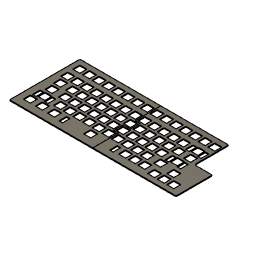
explore-rev3-plate-v1_full (Autodesk Fusion 360 design; units mm, degrees)
Autodesk Fusion 360 part; units mm, degrees
(part 1 of 4)
sketch "Sketch1" plane through (0, 0, 0) normal (0, 1, 0) x (1, 0, 0)
  line L0 (153.7375, -53.475) -> (166.7375, -53.475)
  line L1 (224.675, -92.075) -> (224.675, -105.075)
  line L2 (220.4125, -110.625) -> (233.4125, -110.625)
  line L3 (220.4125, -124.625) -> (233.4125, -124.625)
  line L4 (201.3625, -124.625) -> (214.3625, -124.625)
  line L5 (200.8625, -111.125) -> (200.8625, -124.125)
  line L6 (205.625, -92.075) -> (205.625, -105.075)
  line L7 (187.075, -91.575) -> (200.075, -91.575)
  arc A0 (201.3625, -110.625) -> (200.8625, -111.125) centre (201.3625, -111.125) ccw
  line L8 (219.625, -92.075) -> (219.625, -105.075)
  arc A1 (224.675, -105.075) -> (225.175, -105.575) centre (225.175, -105.075) ccw
  arc A2 (219.9125, -124.125) -> (220.4125, -124.625) centre (220.4125, -124.125) ccw
  line L9 (219.9125, -111.125) -> (219.9125, -124.125)
  line L10 (200.575, -92.075) -> (200.575, -105.075)
  line L11 (196.6, -72.525) -> (209.6, -72.525)
  line L12 (187.075, -105.575) -> (200.075, -105.575)
  line L13 (196.6, -86.525) -> (209.6, -86.525)
  line L14 (191.8375, -67.475) -> (204.8375, -67.475)
  line L15 (168.025, -91.575) -> (181.025, -91.575)
  arc A3 (172, -73.025) -> (171.5, -72.525) centre (171.5, -73.025) ccw
  arc A4 (166.7375, -67.475) -> (167.2375, -66.975) centre (166.7375, -66.975) ccw
  line L16 (177.55, -72.525) -> (190.55, -72.525)
  arc A5 (177.55, -72.525) -> (177.05, -73.025) centre (177.55, -73.025) ccw
  arc A6 (185.7875, -67.475) -> (186.2875, -66.975) centre (185.7875, -66.975) ccw
  arc A7 (171.5, -86.525) -> (172, -86.025) centre (171.5, -86.025) ccw
  arc A8 (196.6, -72.525) -> (196.1, -73.025) centre (196.6, -73.025) ccw
  line L17 (177.05, -73.025) -> (177.05, -86.025)
  arc A9 (191.3375, -66.975) -> (191.8375, -67.475) centre (191.8375, -66.975) ccw
  arc A10 (225.175, -91.575) -> (224.675, -92.075) centre (225.175, -92.075) ccw
  line L18 (215.65, -86.525) -> (228.65, -86.525)
  arc A11 (209.6, -86.525) -> (210.1, -86.025) centre (209.6, -86.025) ccw
  arc A12 (210.3875, -66.975) -> (210.8875, -67.475) centre (210.8875, -66.975) ccw
  arc A13 (215.15, -86.025) -> (215.65, -86.525) centre (215.65, -86.025) ccw
  arc A14 (200.575, -92.075) -> (200.075, -91.575) centre (200.075, -92.075) ccw
  arc A15 (215.65, -72.525) -> (215.15, -73.025) centre (215.65, -73.025) ccw
  line L19 (210.1, -73.025) -> (210.1, -86.025)
  line L20 (158.5, -72.525) -> (171.5, -72.525)
  arc A16 (234.2, -86.025) -> (234.7, -86.525) centre (234.7, -86.025) ccw
  line L21 (158.5, -86.525) -> (171.5, -86.525)
  arc A17 (162.475, -92.075) -> (161.975, -91.575) centre (161.975, -92.075) ccw
  arc A18 (233.9125, -11.1125) -> (233.4125, -10.6125) centre (233.4125, -11.1125) ccw
  arc A19 (214.8625, -34.925) -> (214.3625, -34.425) centre (214.3625, -34.925) ccw
  arc A20 (233.4125, -24.6125) -> (233.9125, -24.1125) centre (233.4125, -24.1125) ccw
  line L22 (195.8125, -11.1125) -> (195.8125, -24.1125)
  line L23 (233.9125, -11.1125) -> (233.9125, -24.1125)
  arc A21 (195.8125, -34.925) -> (195.3125, -34.425) centre (195.3125, -34.925) ccw
  line L24 (201.3625, -34.425) -> (214.3625, -34.425)
  line L25 (214.8625, -11.1125) -> (214.8625, -24.1125)
  arc A22 (214.8625, -11.1125) -> (214.3625, -10.6125) centre (214.3625, -11.1125) ccw
  arc A23 (200.8625, -24.1125) -> (201.3625, -24.6125) centre (201.3625, -24.1125) ccw
  arc A24 (220.4125, -10.6125) -> (219.9125, -11.1125) centre (220.4125, -11.1125) ccw
  line L26 (214.8625, -34.925) -> (214.8625, -47.925)
  line L27 (195.8125, -34.925) -> (195.8125, -47.925)
  line L28 (219.9125, -34.925) -> (219.9125, -47.925)
  line L29 (200.8625, -34.925) -> (200.8625, -47.925)
  line L30 (233.9125, -34.925) -> (233.9125, -47.925)
  arc A25 (205.625, -105.075) -> (206.125, -105.575) centre (206.125, -105.075) ccw
  line L31 (201.3625, -110.625) -> (214.3625, -110.625)
  line L32 (233.9125, -111.125) -> (233.9125, -124.125)
  line L33 (214.8625, -111.125) -> (214.8625, -124.125)
  arc A26 (214.3625, -124.625) -> (214.8625, -124.125) centre (214.3625, -124.125) ccw
  line L34 (206.125, -105.575) -> (219.125, -105.575)
  arc A27 (219.125, -105.575) -> (219.625, -105.075) centre (219.125, -105.075) ccw
  arc A28 (233.9125, -111.125) -> (233.4125, -110.625) centre (233.4125, -111.125) ccw
  arc A29 (200.8625, -124.125) -> (201.3625, -124.625) centre (201.3625, -124.125) ccw
  arc A30 (200.075, -105.575) -> (200.575, -105.075) centre (200.075, -105.075) ccw
  arc A31 (220.4125, -110.625) -> (219.9125, -111.125) centre (220.4125, -111.125) ccw
  arc A32 (233.4125, -124.625) -> (233.9125, -124.125) centre (233.4125, -124.125) ccw
  arc A33 (214.8625, -111.125) -> (214.3625, -110.625) centre (214.3625, -111.125) ccw
  line L35 (220.4125, -10.6125) -> (233.4125, -10.6125)
  arc A34 (214.3625, -24.6125) -> (214.8625, -24.1125) centre (214.3625, -24.1125) ccw
  arc A35 (219.9125, -24.1125) -> (220.4125, -24.6125) centre (220.4125, -24.1125) ccw
  line L36 (220.4125, -24.6125) -> (233.4125, -24.6125)
  line L37 (201.3625, -24.6125) -> (214.3625, -24.6125)
  arc A36 (201.3625, -34.425) -> (200.8625, -34.925) centre (201.3625, -34.925) ccw
  line L38 (200.8625, -11.1125) -> (200.8625, -24.1125)
  arc A37 (195.8125, -11.1125) -> (195.3125, -10.6125) centre (195.3125, -11.1125) ccw
  line L39 (201.3625, -10.6125) -> (214.3625, -10.6125)
  line L40 (220.4125, -34.425) -> (233.4125, -34.425)
  arc A38 (233.9125, -34.925) -> (233.4125, -34.425) centre (233.4125, -34.925) ccw
  line L41 (219.9125, -11.1125) -> (219.9125, -24.1125)
  arc A39 (201.3625, -10.6125) -> (200.8625, -11.1125) centre (201.3625, -11.1125) ccw
  arc A40 (220.4125, -34.425) -> (219.9125, -34.925) centre (220.4125, -34.925) ccw
  arc A41 (195.3125, -24.6125) -> (195.8125, -24.1125) centre (195.3125, -24.1125) ccw
  arc A42 (276.775, -115.8875) -> (276.275, -115.3875) centre (276.275, -115.8875) ccw
  line L42 (281.825, -115.8875) -> (281.825, -128.8875)
  arc A43 (143.425, -92.075) -> (142.925, -91.575) centre (142.925, -92.075) ccw
  line L43 (18.0063, -86.525) -> (31.0063, -86.525)
  arc A44 (10.8625, -10.6125) -> (10.3625, -11.1125) centre (10.8625, -11.1125) ccw
  arc A45 (29.9125, -10.6125) -> (29.4125, -11.1125) centre (29.9125, -11.1125) ccw
  arc A46 (148.975, -91.575) -> (148.475, -92.075) centre (148.975, -92.075) ccw
  arc A47 (10.3625, -24.1125) -> (10.8625, -24.6125) centre (10.8625, -24.1125) ccw
  arc A48 (42.9125, -24.6125) -> (43.4125, -24.1125) centre (42.9125, -24.1125) ccw
  line L44 (29.4125, -34.925) -> (29.4125, -47.925)
  line L45 (14.3308, -92.575) -> (20.3308, -92.575)
  arc A49 (152.95, -73.025) -> (152.45, -72.525) centre (152.45, -73.025) ccw
  line L46 (29.9125, -34.425) -> (42.9125, -34.425)
  line L47 (314.875, -115.8875) -> (314.875, -128.8875)
  line L48 (86.5625, -11.1125) -> (86.5625, -24.1125)
  arc A50 (13.8308, -107.075) -> (14.3308, -107.575) centre (14.3308, -107.075) ccw
  arc A51 (124.375, -92.075) -> (123.875, -91.575) centre (123.875, -92.075) ccw
  line L49 (10.8625, -10.6125) -> (23.8625, -10.6125)
  arc A52 (38.9375, -66.975) -> (39.4375, -67.475) centre (39.4375, -66.975) ccw
  line L50 (36.5563, -111.125) -> (36.5563, -124.125)
  line L51 (29.9125, -24.6125) -> (42.9125, -24.6125)
  line L52 (29.9125, -10.6125) -> (42.9125, -10.6125)
  arc A53 (115.1375, -66.975) -> (115.6375, -67.475) centre (115.6375, -66.975) ccw
  arc A54 (10.8625, -34.425) -> (10.3625, -34.925) centre (10.8625, -34.925) ccw
  line L53 (91.825, -105.575) -> (104.825, -105.575)
  arc A55 (29.9125, -34.425) -> (29.4125, -34.925) centre (29.9125, -34.925) ccw
  arc A56 (109.5875, -67.475) -> (110.0875, -66.975) centre (109.5875, -66.975) ccw
  arc A57 (24.3625, -34.925) -> (23.8625, -34.425) centre (23.8625, -34.925) ccw
  line L54 (53.725, -105.575) -> (66.725, -105.575)
  arc A58 (50.0563, -124.625) -> (50.5563, -124.125) centre (50.0563, -124.125) ccw
  line L55 (43.4125, -34.925) -> (43.4125, -47.925)
  arc A59 (20.8308, -93.075) -> (20.3308, -92.575) centre (20.3308, -93.075) ccw
  arc A60 (110.0875, -53.975) -> (109.5875, -53.475) centre (109.5875, -53.975) ccw
  arc A61 (48.9625, -34.425) -> (48.4625, -34.925) centre (48.9625, -34.925) ccw
  arc A62 (92.3063, -112.125) -> (91.8063, -111.625) centre (91.8063, -112.125) ccw
  arc A63 (48.9625, -10.6125) -> (48.4625, -11.1125) centre (48.9625, -11.1125) ccw
  arc A64 (43.7, -86.025) -> (44.2, -86.525) centre (44.2, -86.025) ccw
  arc A65 (134.1875, -66.975) -> (134.6875, -67.475) centre (134.6875, -66.975) ccw
  arc A66 (43.4125, -11.1125) -> (42.9125, -10.6125) centre (42.9125, -11.1125) ccw
  arc A67 (147.6875, -67.475) -> (148.1875, -66.975) centre (147.6875, -66.975) ccw
  line L56 (120.4, -86.525) -> (133.4, -86.525)
  line L57 (29.4125, -11.1125) -> (29.4125, -24.1125)
  arc A68 (114.35, -86.525) -> (114.85, -86.025) centre (114.35, -86.025) ccw
  arc A69 (96.0875, -66.975) -> (96.5875, -67.475) centre (96.5875, -66.975) ccw
  arc A70 (138.95, -86.025) -> (139.45, -86.525) centre (139.45, -86.025) ccw
  line L58 (48.4625, -11.1125) -> (48.4625, -24.1125)
  arc A71 (20.3308, -107.575) -> (20.8308, -107.075) centre (20.3308, -107.075) ccw
  line L59 (14.3308, -107.575) -> (20.3308, -107.575)
  arc A72 (26.2438, -124.625) -> (26.7438, -124.125) centre (26.2438, -124.125) ccw
  line L60 (13.2438, -110.625) -> (26.2438, -110.625)
  line L61 (22.7688, -91.575) -> (35.7688, -91.575)
  arc A73 (43.4125, -34.925) -> (42.9125, -34.425) centre (42.9125, -34.925) ccw
  arc A74 (31.5063, -73.025) -> (31.0063, -72.525) centre (31.0063, -73.025) ccw
  arc A75 (36.2688, -92.075) -> (35.7688, -91.575) centre (35.7688, -92.075) ccw
  line L62 (85.3063, -112.125) -> (85.3063, -126.125)
  arc A76 (314.875, -115.8875) -> (314.375, -115.3875) centre (314.375, -115.8875) ccw
  line L63 (50.5563, -111.125) -> (50.5563, -124.125)
  arc A77 (153.2375, -66.975) -> (153.7375, -67.475) centre (153.7375, -66.975) ccw
  arc A78 (91.325, -105.075) -> (91.825, -105.575) centre (91.825, -105.075) ccw
  line L64 (24.3625, -11.1125) -> (24.3625, -24.1125)
  arc A79 (18.0063, -72.525) -> (17.5063, -73.025) centre (18.0063, -73.025) ccw
  arc A80 (12.7438, -124.125) -> (13.2438, -124.625) centre (13.2438, -124.125) ccw
  line L65 (12.7438, -111.125) -> (12.7438, -124.125)
  line L66 (114.85, -73.025) -> (114.85, -86.025)
  line L67 (272.8, -67.475) -> (285.8, -67.475)
  arc A81 (119.6125, -11.1125) -> (119.1125, -10.6125) centre (119.1125, -11.1125) ccw
  arc A82 (277.0625, -24.1125) -> (277.5625, -24.6125) centre (277.5625, -24.1125) ccw
  arc A83 (266.0995, -35.925) -> (265.5995, -35.425) centre (265.5995, -35.925) ccw
  line L68 (53.225, -92.075) -> (53.225, -105.075)
  line L69 (281.0943, -73.525) -> (287.0943, -73.525)
  line L70 (91.325, -92.075) -> (91.325, -105.075)
  arc A84 (281.0943, -73.525) -> (280.5943, -74.025) centre (281.0943, -74.025) ccw
  arc A85 (272.3, -66.975) -> (272.8, -67.475) centre (272.8, -66.975) ccw
  line L71 (277.0625, -11.1125) -> (277.0625, -24.1125)
  line L72 (152.95, -73.025) -> (152.95, -86.025)
  arc A86 (157.2125, -24.6125) -> (157.7125, -24.1125) centre (157.2125, -24.1125) ccw
  arc A87 (290.5625, -24.6125) -> (291.0625, -24.1125) centre (290.5625, -24.1125) ccw
  arc A88 (87.0625, -34.425) -> (86.5625, -34.925) centre (87.0625, -34.925) ccw
  arc A89 (128.6375, -67.475) -> (129.1375, -66.975) centre (128.6375, -66.975) ccw
  arc A90 (15.625, -53.475) -> (15.125, -53.975) centre (15.625, -53.975) ccw
  line L73 (250.8688, -92.075) -> (250.8688, -105.075)
  arc A91 (285.8, -67.475) -> (286.3, -66.975) centre (285.8, -66.975) ccw
  line L74 (279.1563, -73.025) -> (279.1563, -86.025)
  line L75 (272.0125, -11.1125) -> (272.0125, -24.1125)
  arc A92 (272.0125, -11.1125) -> (271.5125, -10.6125) centre (271.5125, -11.1125) ccw
  line L76 (144.2125, -10.6125) -> (157.2125, -10.6125)
  line L77 (131.8063, -111.125) -> (131.8063, -124.125)
  line L78 (287.5943, -74.025) -> (287.5943, -88.025)
  arc A93 (158.5, -72.525) -> (158, -73.025) centre (158.5, -73.025) ccw
  line L79 (67.5125, -11.1125) -> (67.5125, -24.1125)
  line L80 (125.1625, -24.6125) -> (138.1625, -24.6125)
  arc A94 (158, -86.025) -> (158.5, -86.525) centre (158.5, -86.025) ccw
  line L81 (96.5875, -53.475) -> (109.5875, -53.475)
  line L82 (119.6125, -11.1125) -> (119.6125, -24.1125)
  line L83 (81.5125, -11.1125) -> (81.5125, -24.1125)
  line L84 (145.8063, -111.125) -> (145.8063, -124.125)
  arc A95 (29.125, -53.975) -> (28.625, -53.475) centre (28.625, -53.975) ccw
  line L85 (280.5943, -74.025) -> (280.5943, -88.025)
  line L86 (124.6625, -11.1125) -> (124.6625, -24.1125)
  arc A96 (278.6563, -86.525) -> (279.1563, -86.025) centre (278.6563, -86.025) ccw
  line L87 (68.0125, -10.6125) -> (81.0125, -10.6125)
  line L88 (44.7068, -93.075) -> (44.7068, -107.075)
  line L89 (132.3063, -110.625) -> (145.3063, -110.625)
  arc A97 (124.6625, -24.1125) -> (125.1625, -24.6125) centre (125.1625, -24.1125) ccw
  line L90 (39.4375, -53.475) -> (52.4375, -53.475)
  arc A98 (279.1563, -73.025) -> (278.6563, -72.525) centre (278.6563, -73.025) ccw
  arc A99 (138.6625, -34.925) -> (138.1625, -34.425) centre (138.1625, -34.925) ccw
  arc A100 (23.8625, -48.425) -> (24.3625, -47.925) centre (23.8625, -47.925) ccw
  line L91 (72.275, -92.075) -> (72.275, -105.075)
  arc A101 (289.9755, -35.925) -> (289.4755, -35.425) centre (289.4755, -35.925) ccw
  arc A102 (100.0625, -48.425) -> (100.5625, -47.925) centre (100.0625, -47.925) ccw
  line L92 (125.1625, -10.6125) -> (138.1625, -10.6125)
  arc A103 (106.1125, -10.6125) -> (105.6125, -11.1125) centre (106.1125, -11.1125) ccw
  arc A104 (119.1125, -24.6125) -> (119.6125, -24.1125) centre (119.1125, -24.1125) ccw
  line L93 (281.825, -96.8375) -> (281.825, -109.8375)
  line L94 (87.0625, -48.425) -> (100.0625, -48.425)
  line L95 (129.925, -105.575) -> (142.925, -105.575)
  arc A105 (100.5625, -34.925) -> (100.0625, -34.425) centre (100.0625, -34.925) ccw
  line L96 (110.375, -92.075) -> (110.375, -105.075)
  arc A106 (115.6375, -53.475) -> (115.1375, -53.975) centre (115.6375, -53.975) ccw
  line L97 (105.6125, -34.925) -> (105.6125, -47.925)
  arc A107 (157.7125, -11.1125) -> (157.2125, -10.6125) centre (157.2125, -11.1125) ccw
  line L98 (143.425, -92.075) -> (143.425, -105.075)
  arc A108 (280.5943, -88.025) -> (281.0943, -88.525) centre (281.0943, -88.025) ccw
  arc A109 (287.5943, -74.025) -> (287.0943, -73.525) centre (287.0943, -74.025) ccw
  line L99 (295.825, -96.8375) -> (295.825, -109.8375)
  arc A110 (144.2125, -34.425) -> (143.7125, -34.925) centre (144.2125, -34.925) ccw
  arc A111 (133.4, -86.525) -> (133.9, -86.025) centre (133.4, -86.025) ccw
  arc A112 (39.4375, -53.475) -> (38.9375, -53.975) centre (39.4375, -53.975) ccw
  arc A113 (129.425, -105.075) -> (129.925, -105.575) centre (129.925, -105.075) ccw
  line L100 (282.325, -129.3875) -> (295.325, -129.3875)
  arc A114 (87.0625, -10.6125) -> (86.5625, -11.1125) centre (87.0625, -11.1125) ccw
  line L101 (10.8625, -48.425) -> (23.8625, -48.425)
  line L102 (138.6625, -34.925) -> (138.6625, -47.925)
  line L103 (20.8308, -93.075) -> (20.8308, -107.075)
  arc A115 (86.5625, -24.1125) -> (87.0625, -24.6125) centre (87.0625, -24.1125) ccw
  arc A116 (42.9125, -48.425) -> (43.4125, -47.925) centre (42.9125, -47.925) ccw
  line L104 (129.925, -91.575) -> (142.925, -91.575)
  arc A117 (100.5625, -11.1125) -> (100.0625, -10.6125) centre (100.0625, -11.1125) ccw
  line L105 (48.4625, -34.925) -> (48.4625, -47.925)
  line L106 (282.325, -110.3375) -> (295.325, -110.3375)
  line L107 (157.7125, -11.1125) -> (157.7125, -24.1125)
  arc A118 (287.0943, -88.525) -> (287.5943, -88.025) centre (287.0943, -88.025) ccw
  line L108 (300.875, -115.8875) -> (300.875, -128.8875)
  arc A119 (125.1625, -10.6125) -> (124.6625, -11.1125) centre (125.1625, -11.1125) ccw
  line L109 (133.9, -73.025) -> (133.9, -86.025)
  arc A120 (132.3063, -110.625) -> (131.8063, -111.125) centre (132.3063, -111.125) ccw
  arc A121 (10.3625, -47.925) -> (10.8625, -48.425) centre (10.8625, -47.925) ccw
  arc A122 (48.4625, -47.925) -> (48.9625, -48.425) centre (48.9625, -47.925) ccw
  line L110 (138.6625, -11.1125) -> (138.6625, -24.1125)
  arc A123 (133.9, -73.025) -> (133.4, -72.525) centre (133.4, -73.025) ccw
  arc A124 (91.0375, -53.975) -> (90.5375, -53.475) centre (90.5375, -53.975) ccw
  arc A125 (125.1625, -34.425) -> (124.6625, -34.925) centre (125.1625, -34.925) ccw
  line L111 (132.3063, -124.625) -> (145.3063, -124.625)
  line L112 (301.375, -115.3875) -> (314.375, -115.3875)
  line L113 (15.625, -53.475) -> (28.625, -53.475)
  arc A126 (123.875, -105.575) -> (124.375, -105.075) centre (123.875, -105.075) ccw
  arc A127 (96.5875, -53.475) -> (96.0875, -53.975) centre (96.5875, -53.975) ccw
  arc A128 (142.925, -105.575) -> (143.425, -105.075) centre (142.925, -105.075) ccw
  arc A129 (157.7125, -34.925) -> (157.2125, -34.425) centre (157.2125, -34.925) ccw
  line L114 (29.9125, -48.425) -> (42.9125, -48.425)
  line L115 (143.7125, -11.1125) -> (143.7125, -24.1125)
  line L116 (48.9625, -10.6125) -> (61.9625, -10.6125)
  line L117 (281.0943, -88.525) -> (287.0943, -88.525)
  line L118 (100.5625, -11.1125) -> (100.5625, -24.1125)
  line L119 (295.825, -115.8875) -> (295.825, -128.8875)
  arc A130 (314.375, -129.3875) -> (314.875, -128.8875) centre (314.375, -128.8875) ccw
  line L120 (87.0625, -24.6125) -> (100.0625, -24.6125)
  line L121 (119.6125, -34.925) -> (119.6125, -47.925)
  arc A131 (295.325, -110.3375) -> (295.825, -109.8375) centre (295.325, -109.8375) ccw
  line L122 (157.7125, -34.925) -> (157.7125, -47.925)
  arc A132 (144.2125, -10.6125) -> (143.7125, -11.1125) centre (144.2125, -11.1125) ccw
  arc A133 (281.825, -109.8375) -> (282.325, -110.3375) centre (282.325, -109.8375) ccw
  arc A134 (86.5625, -47.925) -> (87.0625, -48.425) centre (87.0625, -47.925) ccw
  line L123 (37.7068, -93.075) -> (37.7068, -107.075)
  line L124 (105.6125, -11.1125) -> (105.6125, -24.1125)
  line L125 (134.6875, -67.475) -> (147.6875, -67.475)
  arc A135 (145.3063, -124.625) -> (145.8063, -124.125) centre (145.3063, -124.125) ccw
  arc A136 (276.275, -129.3875) -> (276.775, -128.8875) centre (276.275, -128.8875) ccw
  line L126 (86.5625, -34.925) -> (86.5625, -47.925)
  arc A137 (145.8063, -111.125) -> (145.3063, -110.625) centre (145.3063, -111.125) ccw
  arc A138 (106.1125, -34.425) -> (105.6125, -34.925) centre (106.1125, -34.925) ccw
  arc A139 (143.7125, -24.1125) -> (144.2125, -24.6125) centre (144.2125, -24.1125) ccw
  arc A140 (29.4125, -47.925) -> (29.9125, -48.425) centre (29.9125, -47.925) ccw
  arc A141 (295.825, -96.8375) -> (295.325, -96.3375) centre (295.325, -96.8375) ccw
  arc A142 (148.475, -105.075) -> (148.975, -105.575) centre (148.975, -105.075) ccw
  arc A143 (131.8063, -124.125) -> (132.3063, -124.625) centre (132.3063, -124.125) ccw
  line L127 (124.6625, -34.925) -> (124.6625, -47.925)
  line L128 (24.3625, -34.925) -> (24.3625, -47.925)
  line L129 (67.225, -92.075) -> (67.225, -105.075)
  line L130 (139.45, -72.525) -> (152.45, -72.525)
  line L131 (158, -73.025) -> (158, -86.025)
  arc A144 (295.325, -129.3875) -> (295.825, -128.8875) centre (295.325, -128.8875) ccw
  arc A145 (86.275, -92.075) -> (85.775, -91.575) centre (85.775, -92.075) ccw
  arc A146 (105.6125, -24.1125) -> (106.1125, -24.6125) centre (106.1125, -24.1125) ccw
  arc A147 (110.875, -91.575) -> (110.375, -92.075) centre (110.875, -92.075) ccw
  line L132 (85.8063, -111.625) -> (91.8063, -111.625)
  line L133 (100.5625, -34.925) -> (100.5625, -47.925)
  arc A148 (100.0625, -24.6125) -> (100.5625, -24.1125) centre (100.0625, -24.1125) ccw
  arc A149 (120.4, -72.525) -> (119.9, -73.025) centre (120.4, -73.025) ccw
  line L134 (13.8308, -93.075) -> (13.8308, -107.075)
  arc A150 (85.8063, -111.625) -> (85.3063, -112.125) centre (85.8063, -112.125) ccw
  line L135 (85.8063, -126.625) -> (91.8063, -126.625)
  line L136 (301.375, -129.3875) -> (314.375, -129.3875)
  arc A151 (300.875, -128.8875) -> (301.375, -129.3875) centre (301.375, -128.8875) ccw
  arc A152 (23.8625, -24.6125) -> (24.3625, -24.1125) centre (23.8625, -24.1125) ccw
  arc A153 (105.6125, -47.925) -> (106.1125, -48.425) centre (106.1125, -47.925) ccw
  arc A154 (85.3063, -126.125) -> (85.8063, -126.625) centre (85.8063, -126.125) ccw
  arc A155 (295.825, -115.8875) -> (295.325, -115.3875) centre (295.325, -115.8875) ccw
  arc A156 (281.825, -128.8875) -> (282.325, -129.3875) centre (282.325, -128.8875) ccw
  arc A157 (301.375, -115.3875) -> (300.875, -115.8875) centre (301.375, -115.8875) ccw
  arc A158 (110.375, -105.075) -> (110.875, -105.575) centre (110.875, -105.075) ccw
  arc A159 (282.325, -115.3875) -> (281.825, -115.8875) centre (282.325, -115.8875) ccw
  line L137 (22.2688, -92.075) -> (22.2688, -105.075)
  line L138 (36.2688, -92.075) -> (36.2688, -105.075)
  arc A160 (91.8063, -126.625) -> (92.3063, -126.125) centre (91.8063, -126.125) ccw
  arc A161 (104.825, -105.575) -> (105.325, -105.075) centre (104.825, -105.075) ccw
  arc A162 (139.45, -72.525) -> (138.95, -73.025) centre (139.45, -73.025) ccw
  line L139 (10.3625, -34.925) -> (10.3625, -47.925)
  line L140 (92.3063, -112.125) -> (92.3063, -126.125)
  arc A163 (129.925, -91.575) -> (129.425, -92.075) centre (129.925, -92.075) ccw
  line L141 (276.775, -115.8875) -> (276.775, -128.8875)
  arc A164 (85.775, -105.575) -> (86.275, -105.075) centre (85.775, -105.075) ccw
  line L142 (87.0625, -10.6125) -> (100.0625, -10.6125)
  line L143 (143.7125, -34.925) -> (143.7125, -47.925)
  line L144 (87.0625, -34.425) -> (100.0625, -34.425)
  line L145 (282.325, -115.3875) -> (295.325, -115.3875)
  arc A165 (36.5563, -124.125) -> (37.0563, -124.625) centre (37.0563, -124.125) ccw
  arc A166 (119.9, -86.025) -> (120.4, -86.525) centre (120.4, -86.025) ccw
  line L146 (60.8688, -110.625) -> (73.8688, -110.625)
  line L147 (101.35, -72.525) -> (114.35, -72.525)
  line L148 (10.8625, -24.6125) -> (23.8625, -24.6125)
  line L149 (17.5063, -73.025) -> (17.5063, -86.025)
  line L150 (10.3625, -11.1125) -> (10.3625, -24.1125)
  arc A167 (22.2688, -105.075) -> (22.7688, -105.575) centre (22.7688, -105.075) ccw
  line L151 (15.625, -67.475) -> (28.625, -67.475)
  line L152 (31.5063, -73.025) -> (31.5063, -86.025)
  arc A168 (15.125, -66.975) -> (15.625, -67.475) centre (15.625, -66.975) ccw
  arc A169 (44.2, -72.525) -> (43.7, -73.025) centre (44.2, -73.025) ccw
  line L153 (43.4125, -11.1125) -> (43.4125, -24.1125)
  arc A170 (44.2068, -107.575) -> (44.7068, -107.075) centre (44.2068, -107.075) ccw
  arc A171 (38.2068, -92.575) -> (37.7068, -93.075) centre (38.2068, -93.075) ccw
  arc A172 (91.825, -91.575) -> (91.325, -92.075) centre (91.825, -92.075) ccw
  arc A173 (60.3688, -124.125) -> (60.8688, -124.625) centre (60.8688, -124.125) ccw
  line L154 (101.35, -86.525) -> (114.35, -86.525)
  arc A174 (48.4625, -24.1125) -> (48.9625, -24.6125) centre (48.9625, -24.1125) ccw
  line L155 (96.5875, -67.475) -> (109.5875, -67.475)
  arc A175 (105.325, -92.075) -> (104.825, -91.575) centre (104.825, -92.075) ccw
  arc A176 (37.0563, -110.625) -> (36.5563, -111.125) centre (37.0563, -111.125) ccw
  line L156 (18.0063, -72.525) -> (31.0063, -72.525)
  arc A177 (35.7688, -105.575) -> (36.2688, -105.075) centre (35.7688, -105.075) ccw
  line L157 (60.3688, -111.125) -> (60.3688, -124.125)
  arc A178 (24.3625, -11.1125) -> (23.8625, -10.6125) centre (23.8625, -11.1125) ccw
  arc A179 (26.7438, -111.125) -> (26.2438, -110.625) centre (26.2438, -111.125) ccw
  arc A180 (29.4125, -24.1125) -> (29.9125, -24.6125) centre (29.9125, -24.1125) ccw
  arc A181 (13.2438, -110.625) -> (12.7438, -111.125) centre (13.2438, -111.125) ccw
  arc A182 (31.0063, -86.525) -> (31.5063, -86.025) centre (31.0063, -86.025) ccw
  line L158 (26.7438, -111.125) -> (26.7438, -124.125)
  arc A183 (14.3308, -92.575) -> (13.8308, -93.075) centre (14.3308, -93.075) ccw
  line L159 (38.2068, -107.575) -> (44.2068, -107.575)
  line L160 (43.7, -73.025) -> (43.7, -86.025)
  arc A184 (44.7068, -93.075) -> (44.2068, -92.575) centre (44.2068, -93.075) ccw
  line L161 (38.2068, -92.575) -> (44.2068, -92.575)
  arc A185 (50.5563, -111.125) -> (50.0563, -110.625) centre (50.0563, -111.125) ccw
  arc A186 (90.5375, -67.475) -> (91.0375, -66.975) centre (90.5375, -66.975) ccw
  line L162 (22.7688, -105.575) -> (35.7688, -105.575)
  arc A187 (17.5063, -86.025) -> (18.0063, -86.525) centre (18.0063, -86.025) ccw
  arc A188 (72.275, -105.075) -> (72.775, -105.575) centre (72.775, -105.075) ccw
  arc A189 (60.8688, -110.625) -> (60.3688, -111.125) centre (60.8688, -111.125) ccw
  arc A190 (53.225, -105.075) -> (53.725, -105.575) centre (53.725, -105.075) ccw
  arc A191 (74.3688, -111.125) -> (73.8688, -110.625) centre (73.8688, -111.125) ccw
  arc A192 (28.625, -67.475) -> (29.125, -66.975) centre (28.625, -66.975) ccw
  arc A193 (22.7688, -91.575) -> (22.2688, -92.075) centre (22.7688, -92.075) ccw
  arc A194 (101.35, -72.525) -> (100.85, -73.025) centre (101.35, -73.025) ccw
  line L163 (95.8, -73.025) -> (95.8, -86.025)
  line L164 (100.85, -73.025) -> (100.85, -86.025)
  arc A195 (114.85, -73.025) -> (114.35, -72.525) centre (114.35, -73.025) ccw
  arc A196 (66.725, -105.575) -> (67.225, -105.075) centre (66.725, -105.075) ccw
  arc A197 (73.8688, -124.625) -> (74.3688, -124.125) centre (73.8688, -124.125) ccw
  line L165 (91.825, -91.575) -> (104.825, -91.575)
  line L166 (60.8688, -124.625) -> (73.8688, -124.625)
  line L167 (13.2438, -124.625) -> (26.2438, -124.625)
  arc A198 (95.3, -86.525) -> (95.8, -86.025) centre (95.3, -86.025) ccw
  arc A199 (95.8, -73.025) -> (95.3, -72.525) centre (95.3, -73.025) ccw
  line L168 (10.8625, -34.425) -> (23.8625, -34.425)
  arc A200 (37.7068, -107.075) -> (38.2068, -107.575) centre (38.2068, -107.075) ccw
  line L169 (74.3688, -111.125) -> (74.3688, -124.125)
  arc A201 (100.85, -86.025) -> (101.35, -86.525) centre (101.35, -86.025) ccw
  line L170 (210.8875, -53.475) -> (223.8875, -53.475)
  line L171 (220.4125, -48.425) -> (233.4125, -48.425)
  arc A202 (195.3125, -48.425) -> (195.8125, -47.925) centre (195.3125, -47.925) ccw
  arc A203 (224.3875, -53.975) -> (223.8875, -53.475) centre (223.8875, -53.975) ccw
  arc A204 (229.9375, -53.475) -> (229.4375, -53.975) centre (229.9375, -53.975) ccw
  arc A205 (200.8625, -47.925) -> (201.3625, -48.425) centre (201.3625, -47.925) ccw
  arc A206 (219.9125, -47.925) -> (220.4125, -48.425) centre (220.4125, -47.925) ccw
  arc A207 (210.8875, -53.475) -> (210.3875, -53.975) centre (210.8875, -53.975) ccw
  arc A208 (205.3375, -53.975) -> (204.8375, -53.475) centre (204.8375, -53.975) ccw
  arc A209 (214.3625, -48.425) -> (214.8625, -47.925) centre (214.3625, -47.925) ccw
  line L172 (148.975, -91.575) -> (161.975, -91.575)
  arc A210 (233.4125, -48.425) -> (233.9125, -47.925) centre (233.4125, -47.925) ccw
  line L173 (201.3625, -48.425) -> (214.3625, -48.425)
  arc A211 (185.8063, -111.625) -> (185.3063, -112.125) centre (185.8063, -112.125) ccw
  arc A212 (167.525, -105.075) -> (168.025, -105.575) centre (168.025, -105.075) ccw
  line L174 (185.3063, -112.125) -> (185.3063, -126.125)
  arc A213 (192.3063, -112.125) -> (191.8063, -111.625) centre (191.8063, -112.125) ccw
  line L175 (185.8063, -126.625) -> (191.8063, -126.625)
  line L176 (268.0375, -34.425) -> (281.0375, -34.425)
  arc A214 (57.7, -73.025) -> (57.2, -72.525) centre (57.2, -73.025) ccw
  arc A215 (282.325, -96.3375) -> (281.825, -96.8375) centre (282.325, -96.8375) ccw
  arc A216 (81.0125, -24.6125) -> (81.5125, -24.1125) centre (81.0125, -24.1125) ccw
  arc A217 (238.9625, -124.125) -> (239.4625, -124.625) centre (239.4625, -124.125) ccw
  line L177 (282.325, -96.3375) -> (295.325, -96.3375)
  line L178 (105.325, -92.075) -> (105.325, -105.075)
  line L179 (252.9625, -34.925) -> (252.9625, -47.925)
  arc A218 (239.4625, -110.625) -> (238.9625, -111.125) centre (239.4625, -111.125) ccw
  line L180 (81.5125, -34.925) -> (81.5125, -47.925)
  arc A219 (252.4625, -124.625) -> (252.9625, -124.125) centre (252.4625, -124.125) ccw
  line L181 (239.4625, -110.625) -> (252.4625, -110.625)
  line L182 (129.425, -92.075) -> (129.425, -105.075)
  arc A220 (67.5125, -47.925) -> (68.0125, -48.425) centre (68.0125, -47.925) ccw
  line L183 (239.4625, -124.625) -> (252.4625, -124.625)
  arc A221 (77.5375, -53.475) -> (77.0375, -53.975) centre (77.5375, -53.975) ccw
  line L184 (238.9625, -111.125) -> (238.9625, -124.125)
  arc A222 (81.8, -86.025) -> (82.3, -86.525) centre (82.3, -86.025) ccw
  line L185 (81.8, -73.025) -> (81.8, -86.025)
  line L186 (48.9625, -24.6125) -> (61.9625, -24.6125)
  arc A223 (61.9625, -24.6125) -> (62.4625, -24.1125) centre (61.9625, -24.1125) ccw
  arc A224 (138.6625, -11.1125) -> (138.1625, -10.6125) centre (138.1625, -11.1125) ccw
  line L187 (138.95, -73.025) -> (138.95, -86.025)
  line L188 (264.8688, -92.075) -> (264.8688, -105.075)
  line L189 (48.9625, -48.425) -> (61.9625, -48.425)
  line L190 (277.5625, -10.6125) -> (290.5625, -10.6125)
  arc A225 (68.0125, -10.6125) -> (67.5125, -11.1125) centre (68.0125, -11.1125) ccw
  line L191 (120.4, -72.525) -> (133.4, -72.525)
  arc A226 (119.6125, -34.925) -> (119.1125, -34.425) centre (119.1125, -34.925) ccw
  line L192 (291.0625, -11.1125) -> (291.0625, -24.1125)
  line L193 (238.675, -92.075) -> (238.675, -105.075)
  arc A227 (283.4755, -35.425) -> (282.9755, -35.925) centre (283.4755, -35.925) ccw
  arc A228 (252.9625, -111.125) -> (252.4625, -110.625) centre (252.4625, -111.125) ccw
  line L194 (44.2, -86.525) -> (57.2, -86.525)
  line L195 (148.475, -92.075) -> (148.475, -105.075)
  line L196 (277.5625, -24.6125) -> (290.5625, -24.6125)
  arc A229 (63.25, -72.525) -> (62.75, -73.025) centre (63.25, -73.025) ccw
  line L197 (139.45, -86.525) -> (152.45, -86.525)
  line L198 (48.9625, -34.425) -> (61.9625, -34.425)
  line L199 (144.2125, -34.425) -> (157.2125, -34.425)
  arc A230 (238.175, -105.575) -> (238.675, -105.075) centre (238.175, -105.075) ccw
  line L200 (252.9625, -111.125) -> (252.9625, -124.125)
  arc A231 (277.5625, -10.6125) -> (277.0625, -11.1125) centre (277.5625, -11.1125) ccw
  arc A232 (271.5125, -24.6125) -> (272.0125, -24.1125) centre (271.5125, -24.1125) ccw
  line L201 (281.5375, -34.925) -> (281.5375, -47.925)
  line L202 (124.375, -92.075) -> (124.375, -105.075)
  line L203 (251.3688, -105.575) -> (264.3688, -105.575)
  line L204 (283.4755, -35.425) -> (289.4755, -35.425)
  arc A233 (138.1625, -24.6125) -> (138.6625, -24.1125) centre (138.1625, -24.1125) ccw
  line L205 (115.6375, -53.475) -> (128.6375, -53.475)
  line L206 (119.9, -73.025) -> (119.9, -86.025)
  arc A234 (81.5125, -34.925) -> (81.0125, -34.425) centre (81.0125, -34.925) ccw
  line L207 (68.0125, -34.425) -> (81.0125, -34.425)
  arc A235 (291.0625, -11.1125) -> (290.5625, -10.6125) centre (290.5625, -11.1125) ccw
  arc A236 (68.0125, -34.425) -> (67.5125, -34.925) centre (68.0125, -34.925) ccw
  arc A237 (281.5375, -34.925) -> (281.0375, -34.425) centre (281.0375, -34.925) ccw
  arc A238 (81.0125, -48.425) -> (81.5125, -47.925) centre (81.0125, -47.925) ccw
  arc A239 (81.5125, -11.1125) -> (81.0125, -10.6125) centre (81.0125, -11.1125) ccw
  arc A240 (264.3688, -105.575) -> (264.8688, -105.075) centre (264.3688, -105.075) ccw
  line L208 (144.2125, -24.6125) -> (157.2125, -24.6125)
  arc A241 (61.9625, -48.425) -> (62.4625, -47.925) centre (61.9625, -47.925) ccw
  arc A242 (268.0375, -34.425) -> (267.5375, -34.925) centre (268.0375, -34.925) ccw
  line L209 (125.1625, -34.425) -> (138.1625, -34.425)
  line L210 (172.2875, -53.975) -> (172.2875, -66.975)
  arc A243 (238.675, -92.075) -> (238.175, -91.575) centre (238.175, -92.075) ccw
  arc A244 (251.3688, -91.575) -> (250.8688, -92.075) centre (251.3688, -92.075) ccw
  line L211 (248.9875, -53.475) -> (261.9875, -53.475)
  line L212 (248.9875, -67.475) -> (261.9875, -67.475)
  arc A245 (72.775, -91.575) -> (72.275, -92.075) centre (72.775, -92.075) ccw
  line L213 (153.2375, -53.975) -> (153.2375, -66.975)
  line L214 (15.125, -53.975) -> (15.125, -66.975)
  line L215 (265.6563, -86.525) -> (278.6563, -86.525)
  line L216 (259.5995, -35.425) -> (265.5995, -35.425)
  line L217 (259.5995, -50.425) -> (265.5995, -50.425)
  line L218 (0, -140) -> (0, 0)
  line L219 (256.7183, -74.025) -> (256.7183, -88.025)
  line L220 (239.4625, -48.425) -> (252.4625, -48.425)
  arc A246 (264.8688, -92.075) -> (264.3688, -91.575) centre (264.3688, -92.075) ccw
  line L221 (129.1375, -53.975) -> (129.1375, -66.975)
  line L222 (110.875, -105.575) -> (123.875, -105.575)
  arc A247 (263.2183, -88.525) -> (263.7183, -88.025) centre (263.2183, -88.025) ccw
  line L223 (52.9375, -53.975) -> (52.9375, -66.975)
  arc A248 (263.7183, -74.025) -> (263.2183, -73.525) centre (263.2183, -74.025) ccw
  line L224 (37.0563, -124.625) -> (50.0563, -124.625)
  line L225 (191.3375, -53.975) -> (191.3375, -66.975)
  line L226 (91.0375, -53.975) -> (91.0375, -66.975)
  line L227 (210.3875, -53.975) -> (210.3875, -66.975)
  arc A249 (248.2, -73.025) -> (247.7, -72.525) centre (247.7, -73.025) ccw
  line L228 (77.0375, -53.975) -> (77.0375, -66.975)
  line L229 (96.0875, -53.975) -> (96.0875, -66.975)
  line L230 (258.5125, -24.6125) -> (271.5125, -24.6125)
  line L231 (257.2183, -88.525) -> (263.2183, -88.525)
  line L232 (110.0875, -53.975) -> (110.0875, -66.975)
  line L233 (115.1375, -53.975) -> (115.1375, -66.975)
  line L234 (57.9875, -53.975) -> (57.9875, -66.975)
  line L235 (38.9375, -53.975) -> (38.9375, -66.975)
  arc A250 (248.4875, -66.975) -> (248.9875, -67.475) centre (248.9875, -66.975) ccw
  line L236 (148.1875, -53.975) -> (148.1875, -66.975)
  line L237 (258.5125, -10.6125) -> (271.5125, -10.6125)
  line L238 (71.9875, -53.975) -> (71.9875, -66.975)
  line L239 (205.3375, -53.975) -> (205.3375, -66.975)
  line L240 (134.1875, -53.975) -> (134.1875, -66.975)
  line L241 (224.3875, -53.975) -> (224.3875, -66.975)
  line L242 (229.4375, -53.975) -> (229.4375, -66.975)
  line L243 (257.2183, -73.525) -> (263.2183, -73.525)
  line L244 (29.125, -53.975) -> (29.125, -66.975)
  line L245 (263.275, -115.3875) -> (276.275, -115.3875)
  arc A251 (242.9375, -67.475) -> (243.4375, -66.975) centre (242.9375, -66.975) ccw
  line L246 (265.6563, -72.525) -> (278.6563, -72.525)
  arc A252 (247.7, -86.525) -> (248.2, -86.025) centre (247.7, -86.025) ccw
  arc A253 (252.4625, -48.425) -> (252.9625, -47.925) centre (252.4625, -47.925) ccw
  arc A254 (238.9625, -24.1125) -> (239.4625, -24.6125) centre (239.4625, -24.1125) ccw
  line L247 (106.1125, -34.425) -> (119.1125, -34.425)
  line L248 (263.275, -129.3875) -> (276.275, -129.3875)
  line L249 (248.2, -73.025) -> (248.2, -86.025)
  arc A255 (252.9625, -34.925) -> (252.4625, -34.425) centre (252.4625, -34.925) ccw
  line L250 (258.0125, -11.1125) -> (258.0125, -24.1125)
  arc A256 (289.4755, -50.425) -> (289.9755, -49.925) centre (289.4755, -49.925) ccw
  line L251 (289.9755, -35.925) -> (289.9755, -49.925)
  line L252 (115.6375, -67.475) -> (128.6375, -67.475)
  line L253 (272.8, -53.475) -> (285.8, -53.475)
  line L254 (53.725, -91.575) -> (66.725, -91.575)
  arc A257 (248.9875, -53.475) -> (248.4875, -53.975) centre (248.9875, -53.975) ccw
  arc A258 (239.4625, -10.6125) -> (238.9625, -11.1125) centre (239.4625, -11.1125) ccw
  line L255 (263.7183, -74.025) -> (263.7183, -88.025)
  line L256 (106.1125, -48.425) -> (119.1125, -48.425)
  arc A259 (267.5375, -47.925) -> (268.0375, -48.425) centre (268.0375, -47.925) ccw
  arc A260 (77.0375, -66.975) -> (77.5375, -67.475) centre (77.5375, -66.975) ccw
  line L257 (68.0125, -24.6125) -> (81.0125, -24.6125)
  arc A261 (265.6563, -72.525) -> (265.1563, -73.025) centre (265.6563, -73.025) ccw
  line L258 (106.1125, -24.6125) -> (119.1125, -24.6125)
  line L259 (106.1125, -10.6125) -> (119.1125, -10.6125)
  arc A262 (261.9875, -67.475) -> (262.4875, -66.975) centre (261.9875, -66.975) ccw
  line L260 (134.6875, -53.475) -> (147.6875, -53.475)
  line L261 (110.875, -91.575) -> (123.875, -91.575)
  line L262 (57.7, -73.025) -> (57.7, -86.025)
  arc A263 (129.1375, -53.975) -> (128.6375, -53.475) centre (128.6375, -53.975) ccw
  line L263 (239.4625, -10.6125) -> (252.4625, -10.6125)
  line L264 (251.3688, -91.575) -> (264.3688, -91.575)
  line L265 (238.9625, -34.925) -> (238.9625, -47.925)
  arc A264 (258.0125, -24.1125) -> (258.5125, -24.6125) centre (258.5125, -24.1125) ccw
  arc A265 (67.5125, -24.1125) -> (68.0125, -24.6125) centre (68.0125, -24.1125) ccw
  arc A266 (71.4875, -67.475) -> (71.9875, -66.975) centre (71.4875, -66.975) ccw
  arc A267 (252.4625, -24.6125) -> (252.9625, -24.1125) centre (252.4625, -24.1125) ccw
  arc A268 (134.6875, -53.475) -> (134.1875, -53.975) centre (134.6875, -53.975) ccw
  arc A269 (257.2183, -73.525) -> (256.7183, -74.025) centre (257.2183, -74.025) ccw
  arc A270 (57.2, -86.525) -> (57.7, -86.025) centre (57.2, -86.025) ccw
  arc A271 (76.25, -86.525) -> (76.75, -86.025) centre (76.25, -86.025) ccw
  arc A272 (272.8, -53.475) -> (272.3, -53.975) centre (272.8, -53.975) ccw
  line L266 (58.4875, -67.475) -> (71.4875, -67.475)
  line L267 (144.2125, -48.425) -> (157.2125, -48.425)
  line L268 (252.9625, -11.1125) -> (252.9625, -24.1125)
  arc A273 (281.0375, -48.425) -> (281.5375, -47.925) centre (281.0375, -47.925) ccw
  arc A274 (53.725, -91.575) -> (53.225, -92.075) centre (53.725, -92.075) ccw
  line L269 (283.4755, -50.425) -> (289.4755, -50.425)
  arc A275 (262.4875, -53.975) -> (261.9875, -53.475) centre (261.9875, -53.975) ccw
  line L270 (265.1563, -73.025) -> (265.1563, -86.025)
  line L271 (68.0125, -48.425) -> (81.0125, -48.425)
  arc A276 (265.1563, -86.025) -> (265.6563, -86.525) centre (265.6563, -86.025) ccw
  arc A277 (238.9625, -47.925) -> (239.4625, -48.425) centre (239.4625, -47.925) ccw
  line L272 (239.4625, -34.425) -> (252.4625, -34.425)
  arc A278 (62.4625, -11.1125) -> (61.9625, -10.6125) centre (61.9625, -11.1125) ccw
  arc A279 (57.9875, -66.975) -> (58.4875, -67.475) centre (58.4875, -66.975) ccw
  arc A280 (138.1625, -48.425) -> (138.6625, -47.925) centre (138.1625, -47.925) ccw
  arc A281 (256.7183, -88.025) -> (257.2183, -88.525) centre (257.2183, -88.025) ccw
  line L273 (266.0995, -35.925) -> (266.0995, -49.925)
  arc A282 (52.4375, -67.475) -> (52.9375, -66.975) centre (52.4375, -66.975) ccw
  line L274 (63.25, -72.525) -> (76.25, -72.525)
  arc A283 (157.2125, -48.425) -> (157.7125, -47.925) centre (157.2125, -47.925) ccw
  line L275 (239.4625, -24.6125) -> (252.4625, -24.6125)
  line L276 (238.9625, -11.1125) -> (238.9625, -24.1125)
  arc A284 (282.9755, -49.925) -> (283.4755, -50.425) centre (283.4755, -49.925) ccw
  arc A285 (124.6625, -47.925) -> (125.1625, -48.425) centre (125.1625, -47.925) ccw
  arc A286 (259.5995, -35.425) -> (259.0995, -35.925) centre (259.5995, -35.925) ccw
  line L277 (86.275, -92.075) -> (86.275, -105.075)
  line L278 (268.0375, -48.425) -> (281.0375, -48.425)
  line L279 (67.5125, -34.925) -> (67.5125, -47.925)
  line L280 (63.25, -86.525) -> (76.25, -86.525)
  line L281 (125.1625, -48.425) -> (138.1625, -48.425)
  line L282 (76.75, -73.025) -> (76.75, -86.025)
  arc A287 (82.3, -72.525) -> (81.8, -73.025) centre (82.3, -73.025) ccw
  arc A288 (262.775, -128.8875) -> (263.275, -129.3875) centre (263.275, -128.8875) ccw
  line L283 (58.4875, -53.475) -> (71.4875, -53.475)
  line L284 (44.2, -72.525) -> (57.2, -72.525)
  arc A289 (263.275, -115.3875) -> (262.775, -115.8875) centre (263.275, -115.8875) ccw
  arc A290 (153.7375, -53.475) -> (153.2375, -53.975) centre (153.7375, -53.975) ccw
  line L285 (37.0563, -110.625) -> (50.0563, -110.625)
  arc A291 (148.1875, -53.975) -> (147.6875, -53.475) centre (147.6875, -53.975) ccw
  arc A292 (67.225, -92.075) -> (66.725, -91.575) centre (66.725, -92.075) ccw
  arc A293 (62.4625, -34.925) -> (61.9625, -34.425) centre (61.9625, -34.925) ccw
  arc A294 (250.8688, -105.075) -> (251.3688, -105.575) centre (251.3688, -105.075) ccw
  line L286 (282.9755, -35.925) -> (282.9755, -49.925)
  line L287 (267.5375, -34.925) -> (267.5375, -47.925)
  line L288 (262.775, -115.8875) -> (262.775, -128.8875)
  arc A295 (71.9875, -53.975) -> (71.4875, -53.475) centre (71.4875, -53.975) ccw
  arc A296 (152.45, -86.525) -> (152.95, -86.025) centre (152.45, -86.025) ccw
  line L289 (62.75, -73.025) -> (62.75, -86.025)
  arc A297 (259.0995, -49.925) -> (259.5995, -50.425) centre (259.5995, -49.925) ccw
  arc A298 (52.9375, -53.975) -> (52.4375, -53.475) centre (52.4375, -53.975) ccw
  arc A299 (243.4375, -53.975) -> (242.9375, -53.475) centre (242.9375, -53.975) ccw
  arc A300 (286.3, -53.975) -> (285.8, -53.475) centre (285.8, -53.975) ccw
  line L290 (62.4625, -34.925) -> (62.4625, -47.925)
  arc A301 (119.1125, -48.425) -> (119.6125, -47.925) centre (119.1125, -47.925) ccw
  arc A302 (252.9625, -11.1125) -> (252.4625, -10.6125) centre (252.4625, -11.1125) ccw
  arc A303 (76.75, -73.025) -> (76.25, -72.525) centre (76.25, -73.025) ccw
  line L291 (62.4625, -11.1125) -> (62.4625, -24.1125)
  line L292 (39.4375, -67.475) -> (52.4375, -67.475)
  arc A304 (265.5995, -50.425) -> (266.0995, -49.925) centre (265.5995, -49.925) ccw
  arc A305 (58.4875, -53.475) -> (57.9875, -53.975) centre (58.4875, -53.975) ccw
  arc A306 (258.5125, -10.6125) -> (258.0125, -11.1125) centre (258.5125, -11.1125) ccw
  arc A307 (143.7125, -47.925) -> (144.2125, -48.425) centre (144.2125, -47.925) ccw
  arc A308 (62.75, -86.025) -> (63.25, -86.525) centre (63.25, -86.025) ccw
  arc A309 (239.4625, -34.425) -> (238.9625, -34.925) centre (239.4625, -34.925) ccw
  line L293 (259.0995, -35.925) -> (259.0995, -49.925)
  arc A310 (228.65, -86.525) -> (229.15, -86.025) centre (228.65, -86.025) ccw
  arc A311 (206.125, -91.575) -> (205.625, -92.075) centre (206.125, -92.075) ccw
  arc A312 (229.4375, -66.975) -> (229.9375, -67.475) centre (229.9375, -66.975) ccw
  line L294 (215.15, -73.025) -> (215.15, -86.025)
  arc A313 (223.8875, -67.475) -> (224.3875, -66.975) centre (223.8875, -66.975) ccw
  line L295 (229.15, -73.025) -> (229.15, -86.025)
  arc A314 (234.7, -72.525) -> (234.2, -73.025) centre (234.7, -73.025) ccw
  arc A315 (219.625, -92.075) -> (219.125, -91.575) centre (219.125, -92.075) ccw
  line L296 (215.65, -72.525) -> (228.65, -72.525)
  line L297 (206.125, -91.575) -> (219.125, -91.575)
  line L298 (181.525, -92.075) -> (181.525, -105.075)
  line L299 (168.025, -105.575) -> (181.025, -105.575)
  arc A316 (191.8063, -126.625) -> (192.3063, -126.125) centre (191.8063, -126.125) ccw
  line L300 (192.3063, -112.125) -> (192.3063, -126.125)
  line L301 (162.475, -92.075) -> (162.475, -105.075)
  arc A317 (161.975, -105.575) -> (162.475, -105.075) centre (161.975, -105.075) ccw
  line L302 (167.525, -92.075) -> (167.525, -105.075)
  line L303 (186.575, -92.075) -> (186.575, -105.075)
  arc A318 (185.3063, -126.125) -> (185.8063, -126.625) centre (185.8063, -126.125) ccw
  arc A319 (186.575, -105.075) -> (187.075, -105.575) centre (187.075, -105.075) ccw
  line L304 (185.8063, -111.625) -> (191.8063, -111.625)
  arc A320 (181.025, -105.575) -> (181.525, -105.075) centre (181.025, -105.075) ccw
  arc A321 (176.2625, -24.6125) -> (176.7625, -24.1125) centre (176.2625, -24.1125) ccw
  line L305 (286.3, -53.975) -> (286.3, -66.975)
  line L306 (272.3, -53.975) -> (272.3, -66.975)
  line L307 (234.7, -72.525) -> (247.7, -72.525)
  line L308 (186.2875, -53.975) -> (186.2875, -66.975)
  line L309 (72.775, -105.575) -> (85.775, -105.575)
  line L310 (330, 0) -> (330, -140)
  line L311 (262.4875, -53.975) -> (262.4875, -66.975)
  line L312 (182.3125, -34.425) -> (195.3125, -34.425)
  line L313 (167.2375, -53.975) -> (167.2375, -66.975)
  line L314 (176.7625, -34.925) -> (176.7625, -47.925)
  arc A322 (181.8125, -24.1125) -> (182.3125, -24.6125) centre (182.3125, -24.1125) ccw
  line L315 (77.5375, -67.475) -> (90.5375, -67.475)
  line L316 (182.3125, -10.6125) -> (195.3125, -10.6125)
  line L317 (82.3, -86.525) -> (95.3, -86.525)
  line L318 (191.8375, -53.475) -> (204.8375, -53.475)
  arc A323 (191.8375, -53.475) -> (191.3375, -53.975) centre (191.8375, -53.975) ccw
  line L319 (181.8125, -11.1125) -> (181.8125, -24.1125)
  arc A324 (176.7625, -11.1125) -> (176.2625, -10.6125) centre (176.2625, -11.1125) ccw
  line L320 (182.3125, -24.6125) -> (195.3125, -24.6125)
  line L321 (243.4375, -53.975) -> (243.4375, -66.975)
  line L322 (248.4875, -53.975) -> (248.4875, -66.975)
  line L323 (163.2625, -48.425) -> (176.2625, -48.425)
  line L324 (82.3, -72.525) -> (95.3, -72.525)
  line L325 (72.775, -91.575) -> (85.775, -91.575)
  line L326 (182.3125, -48.425) -> (195.3125, -48.425)
  arc A325 (176.7625, -34.925) -> (176.2625, -34.425) centre (176.2625, -34.925) ccw
  line L327 (176.7625, -11.1125) -> (176.7625, -24.1125)
  arc A326 (167.2375, -53.975) -> (166.7375, -53.475) centre (166.7375, -53.975) ccw
  arc A327 (163.2625, -34.425) -> (162.7625, -34.925) centre (163.2625, -34.925) ccw
  arc A328 (172.7875, -53.475) -> (172.2875, -53.975) centre (172.7875, -53.975) ccw
  line L328 (0, 0) -> (330, 0)
  arc A329 (162.7625, -47.925) -> (163.2625, -48.425) centre (163.2625, -47.925) ccw
  arc A330 (162.7625, -24.1125) -> (163.2625, -24.6125) centre (163.2625, -24.1125) ccw
  line L329 (162.7625, -11.1125) -> (162.7625, -24.1125)
  line L330 (181.8125, -34.925) -> (181.8125, -47.925)
  line L331 (172.7875, -53.475) -> (185.7875, -53.475)
  arc A331 (182.3125, -10.6125) -> (181.8125, -11.1125) centre (182.3125, -11.1125) ccw
  arc A332 (176.2625, -48.425) -> (176.7625, -47.925) centre (176.2625, -47.925) ccw
  arc A333 (186.2875, -53.975) -> (185.7875, -53.475) centre (185.7875, -53.975) ccw
  line L332 (148.975, -105.575) -> (161.975, -105.575)
  line L333 (163.2625, -24.6125) -> (176.2625, -24.6125)
  line L334 (330, -140) -> (0, -140)
  arc A334 (163.2625, -10.6125) -> (162.7625, -11.1125) centre (163.2625, -11.1125) ccw
  line L335 (229.9375, -67.475) -> (242.9375, -67.475)
  line L336 (163.2625, -34.425) -> (176.2625, -34.425)
  line L337 (162.7625, -34.925) -> (162.7625, -47.925)
  line L338 (153.7375, -67.475) -> (166.7375, -67.475)
  line L339 (225.175, -91.575) -> (238.175, -91.575)
  arc A335 (182.3125, -34.425) -> (181.8125, -34.925) centre (182.3125, -34.925) ccw
  line L340 (225.175, -105.575) -> (238.175, -105.575)
  line L341 (234.7, -86.525) -> (247.7, -86.525)
  line L342 (77.5375, -53.475) -> (90.5375, -53.475)
  line L343 (229.9375, -53.475) -> (242.9375, -53.475)
  line L344 (163.2625, -10.6125) -> (176.2625, -10.6125)
  arc A336 (181.8125, -47.925) -> (182.3125, -48.425) centre (182.3125, -47.925) ccw
  arc A337 (191.05, -73.025) -> (190.55, -72.525) centre (190.55, -73.025) ccw
  arc A338 (181.525, -92.075) -> (181.025, -91.575) centre (181.025, -92.075) ccw
  arc A339 (187.075, -91.575) -> (186.575, -92.075) centre (187.075, -92.075) ccw
  arc A340 (172.2875, -66.975) -> (172.7875, -67.475) centre (172.7875, -66.975) ccw
  line L345 (191.05, -73.025) -> (191.05, -86.025)
  line L346 (196.1, -73.025) -> (196.1, -86.025)
  arc A341 (177.05, -86.025) -> (177.55, -86.525) centre (177.55, -86.025) ccw
  arc A342 (196.1, -86.025) -> (196.6, -86.525) centre (196.6, -86.025) ccw
  arc A343 (168.025, -91.575) -> (167.525, -92.075) centre (168.025, -92.075) ccw
  line L347 (172.7875, -67.475) -> (185.7875, -67.475)
  arc A344 (210.1, -73.025) -> (209.6, -72.525) centre (209.6, -73.025) ccw
  arc A345 (204.8375, -67.475) -> (205.3375, -66.975) centre (204.8375, -66.975) ccw
  line L348 (210.8875, -67.475) -> (223.8875, -67.475)
  arc A346 (229.15, -73.025) -> (228.65, -72.525) centre (228.65, -73.025) ccw
  line L349 (234.2, -73.025) -> (234.2, -86.025)
  line L350 (172, -73.025) -> (172, -86.025)
  line L351 (177.55, -86.525) -> (190.55, -86.525)
  arc A347 (190.55, -86.525) -> (191.05, -86.025) centre (190.55, -86.025) ccw
  point P0 (7.8375, -8.0875)
extrude "Extrude1" add sketch "Sketch1" along normal blind 1.5 makes body 1
fillet "Fillet1" radius 3 4 edges at (0, 0.75, 0) (0, 0.75, 140) (330, 0.75, 0) (330, 0.75, 140) on bodies 1